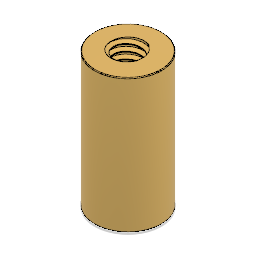
Center Ankle Bushing (Autodesk Fusion 360 design; units mm, degrees)
Autodesk Fusion 360 part; units mm, degrees
sketch "Sketch1" plane through (0, 0, 0) normal (0, 1, 0) x (1, 0, 0)
  circle A0 centre (0, 0) radius 6.35
extrude "Extrude1" add sketch "Sketch1" along normal blind 25.4
fillet "Fillet1" radius 0.127 2 edges at (-5.9203, 25.4, 2.2963) (-5.9203, 0, 2.2963)
sketch "Sketch2" plane through (0, 25.4, 0) normal (0, 1, 0) x (-1, 0, 0)
  circle A0 centre (0, 0) radius 6.223
  circle A1 centre (0, 0) radius 1.27
extrude "Extrude2" cut sketch "Sketch2" against normal blind 25.654 contours A1
thread "Thread1" "ANSI Unified Screw Threads 0.25 1/4-20 UNC 3B" major diameter 6.35 minor diameter 5.1156 pitch 1.27 angle 60 modelled right hand crest width 0.1588 on face at (-1.2637, 8.4667, -0.1265) crest through (-2.5578, 26.1144, 0)
